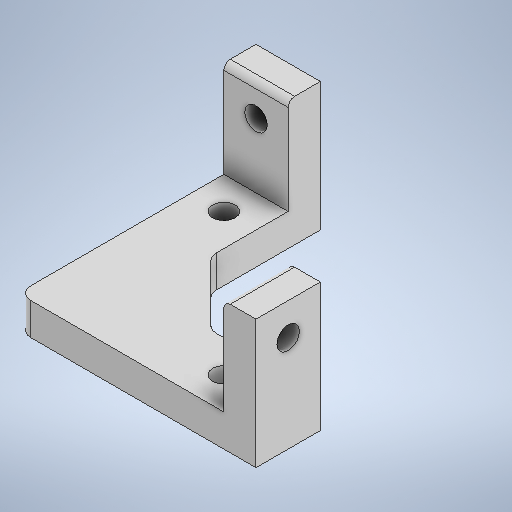
# Autodesk Inventor part: B8-BR-case-bracket
Saved by Autodesk Inventor 2025.2 (Build 292293000, 293)
## iProperties
Created: 2025-11-15
Part Number: B8-BR-case-bracket
Material: 일반
Document SubType Name: Modeling
Designer: RunGeun
Density: 1 g/cm^3
Appearance: 기본값
Author: RunGeun
Autodesk Inventor part; units mm, degrees
ref_plane "YZ Plane" through (0, 0, 0) normal (1, 0, 0) x (0, 1, 0)
ref_plane "XZ Plane" through (0, 0, 0) normal (0, 1, 0) x (-1, 0, 0)
ref_plane "XY Plane" through (0, 0, 0) normal (0, 0, 1) x (1, 0, 0)
sketch "스케치1" plane through (0, 0, 0) normal (0, 1, 0) x (-1, 0, 0)
  circle A0 centre (9.7893, -3.4966) radius 1.75
  circle A1 centre (31.7893, -25.4966) radius 1.75
  line L0 (36.7893, 1.5034) -> (-0.2107, 1.5034)
  line L1 (-0.2107, 1.5034) -> (-0.2107, -8.4966)
  line L2 (26.7893, -35.4966) -> (36.7893, -35.4966)
  line L3 (36.7893, -35.4966) -> (36.7893, 1.5034)
  line L4 (26.7893, -8.4966) -> (-0.2107, -8.4966)
  line L5 (26.7893, -35.4966) -> (26.7893, -8.4966)
  line L6 (26.7893, -35.4966) -> (36.7893, -35.4966)
  line L7 (36.7893, -35.4966) -> (36.7893, -30.4966)
  line L8 (36.7893, -30.4966) -> (26.7893, -30.4966)
  line L9 (26.7893, -30.4966) -> (26.7893, -35.4966)
  line L10 (-0.2107, -8.4966) -> (4.7893, -8.4966)
  line L11 (4.7893, -8.4966) -> (4.7893, 1.5034)
  line L12 (4.7893, 1.5034) -> (-0.2107, 1.5034)
  line L13 (-0.2107, 1.5034) -> (-0.2107, -8.4966)
  point P0 (0, 0)
  dimension "d0" = 3.5
  dimension "d1" = 3.5
  dimension "d2" = 10
  dimension "d3" = 10
  dimension "d4" = 5
  dimension "d5" = 5
  dimension "d6" = 5
  dimension "d7" = 5
  dimension "d8" = 22
  dimension "d9" = 22
  dimension "d10" = 5
  dimension "d11" = 5
  constraints: 28 end point, 6 parallel, 4 horizontal, 3 perpendicular, 2 centre point, 2 point on line
  measures "d0" diameter of A1
  measures "d1" diameter of A0
  measures "d2" distance from line of A1.centre L2
  measures "d3" distance from line of A0.centre L1
  measures "d4" distance from line of A0.centre L0
  measures "d5" distance from line of A0.centre L4
  measures "d6" distance from line of A1.centre L5
  measures "d7" distance from line of A1.centre L3
  measures "d8" horizontal distance of A1.centre A0.centre
  measures "d9" horizontal distance of A0.centre A1.centre
  measures "d10" distance of L7.end L6.end
  measures "d11" distance of L12.end L11.end
extrude "돌출1" add sketch "스케치1" along normal blind 5 contours L3 L8 L5 L4 L11 L0
extrude "돌출2" add sketch "스케치1" along normal blind 20 contours L11 L4 L1 L0 | L3 L2 L5 L8
chamfer "모따기1" distance 10 angle 45 1 edges at (-26.7893, 2.5, -8.4966)
fillet "모깎기1" radius 2 3 edges at (-36.7893, 2.5, 1.5034) (-16.7893, 2.5, -8.4966) (-26.7893, 2.5, -18.4966)
sketch "스케치2" plane through (-4.7893, 5, 1.5034) normal (-1, 0, 0) x (0, 0, 1)
  circle A0 centre (-5, 10) radius 1.75
  line L0 (0, 0) -> (0, 15) projected
  line L1 (-10, 15) -> (0, 15) projected
  point P0 (-1.5034, -5)
  dimension "d20" = 3.5
  dimension "d21" = 5
  dimension "d22" = 5
  constraints: 1 centre point
  measures "d20" diameter of A0
  measures "d21" distance from line of L0 A0.centre
  measures "d22" distance from line of A0.centre L1
extrude "돌출3" cut sketch "스케치2" against normal blind 20
sketch "스케치3" plane through (-36.7893, 5, -30.4966) normal (0, 0, 1) x (1, 0, 0)
  circle A0 centre (5, 10) radius 1.75
  line L0 (10, 0) -> (10, 15) projected
  line L1 (0, 15) -> (10, 15) projected
  point P0 (36.7893, -5)
  dimension "d25" = 3.5
  dimension "d26" = 5
  dimension "d27" = 5
  constraints: 1 centre point
  measures "d25" diameter of A0
  measures "d26" distance from line of A0.centre L0
  measures "d27" distance from line of A0.centre L1
extrude "돌출4" cut sketch "스케치3" against normal blind 20
fillet "모깎기2" radius 1 2 edges at (-31.7893, 20, -30.4966) (-4.7893, 20, -3.4966)
equation "\"d1\" = d0"
equation "\"d3\" = d2"
equation "\"d5\" = d4"
equation "\"d6\" = d4"
equation "\"d7\" = d6"
equation "\"d27\" = d26"
